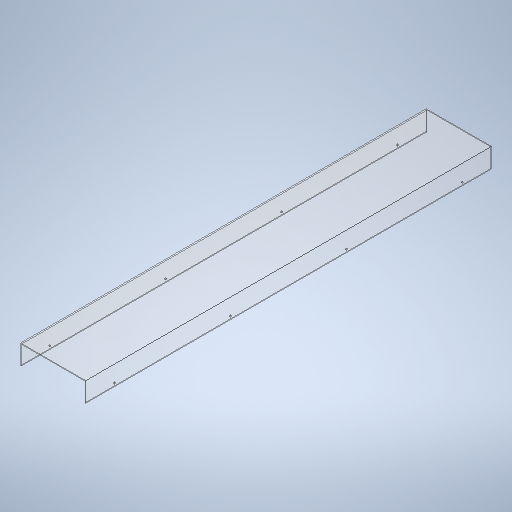
# Autodesk Inventor part: Teste Placa
Saved by Autodesk Inventor 2025.3 (Build 293356030, 356C)
## iProperties
Created: 2025-11-09
Part Number: Teste Placa
Material: Policarbonato, transparente
Document SubType Name: Modeling
Designer: Rubens
Density: 1.2 g/cm^3
Appearance: Policarbonato - Transparente
Author: Rubens
Autodesk Inventor part; units mm, degrees
ref_plane "YZ Plane" through (0, 0, 0) normal (1, 0, 0) x (0, 1, 0)
ref_plane "XZ Plane" through (0, 0, 0) normal (0, 1, 0) x (-1, 0, 0)
ref_plane "XY Plane" through (0, 0, 0) normal (0, 0, 1) x (1, 0, 0)
sketch "Esboço1" plane through (0, 0, 0) normal (0, 0, 1) x (1, 0, 0)
  line L0 (-220.4936, -60.1777) -> (-220.4936, -0.1777)
  line L1 (219.5064, -0.1777) -> (219.5064, -60.1777)
  line L2 (224.5064, -60.1777) -> (224.5064, 4.8223)
  line L3 (-225.4936, 4.8223) -> (-225.4936, -60.1777)
  line L4 (-225.4936, 4.8223) -> (-225.4936, 74.8223)
  line L5 (-225.4936, 74.8223) -> (224.5064, 74.8223)
  line L6 (224.5064, 74.8223) -> (224.5064, 4.8223)
  line L7 (219.5064, -60.1777) -> (219.5064, 4.8223)
  line L8 (219.5064, 4.8223) -> (219.5064, 69.8223)
  line L9 (219.5064, 69.8223) -> (-220.4936, 69.8223)
  line L10 (-220.4936, 69.8223) -> (-220.4936, 4.8223)
  line L11 (-220.4936, 4.8223) -> (-220.4936, -60.1777)
  line L12 (-220.4936, -60.1777) -> (-225.4936, -60.1777)
  line L13 (224.5064, -60.1777) -> (219.5064, -60.1777)
  point P0 (0, 0)
  dimension "d0" = 60
  dimension "d1" = 440
  dimension "d2" = 70
  dimension "d3" = 5
  constraints: 28 end point, 5 perpendicular, 1 collinear, 1 parallel, 1 vertical, 4 other
  measures "d0" distance of L0.start L0.end
  measures "d1" distance of L0.end L1.start
  measures "d2" distance of L3.start L4.end
  measures "d3" distance between parallel lines of L5 L9
extrude "Extrusão1" add sketch "Esboço1" along normal blind 2800
sketch "Esboço2" plane through (224.5064, -60.1777, 0) normal (1, 0, 0) x (0, 0, -1)
  line L0 (0, 0) -> (-2800, 0) projected
  line L1 (0, 0) -> (-2800, 0)
  line L2 (-2800, 0) -> (-2800, 40)
  line L3 (-2800, 40) -> (0, 40)
  line L4 (0, 40) -> (0, 0)
  circle A0 centre (-200, 20) radius 5
  circle A1 centre (-1000, 20) radius 5
  circle A2 centre (-1800, 20) radius 5
  circle A3 centre (-2600, 20) radius 5
  point P0 (0, 60.1777)
  dimension "d6" = 2800
  dimension "d7" = 40
  dimension "d8" = 10
  dimension "d9" = 10
  dimension "d10" = 10
  dimension "d11" = 10
  dimension "d12" = 20
  dimension "d13" = 20
  dimension "d14" = 20
  dimension "d15" = 20
  dimension "d16" = 800
  dimension "d17" = 800
  dimension "d18" = 800
  dimension "d19" = 200
  constraints: 8 end point, 4 centre point, 2 parallel, 1 horizontal, 1 perpendicular
  measures "d6" distance of L2.end L3.end
  measures "d7" distance between parallel lines of L0 L3
  measures "d8" diameter of A0
  measures "d9" diameter of A1
  measures "d10" diameter of A2
  measures "d11" diameter of A3
  measures "d12" distance from line of L3 A3.centre
  measures "d13" distance from line of L3 A2.centre
  measures "d14" distance from line of L3 A1.centre
  measures "d15" distance from line of L3 A0.centre
  measures "d16" distance of A1.centre A0.centre
  measures "d17" distance of A2.centre A1.centre
  measures "d18" distance of A3.centre A2.centre
  measures "d19" distance from line of L4 A0.centre
extrude "Extrusão2" cut sketch "Esboço2" against normal through all contours A0 | A1 | A2 | A3
